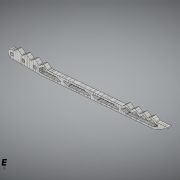
# Autodesk Inventor part: カウンター短
Saved by Autodesk Inventor 2020 (Build 240168000, 168)
## iProperties
Created: 2019-11-14
Part Number: カウンター短
Material: アルミニウム 7075
Document SubType Name: Modeling
Designer: tanjihayato
Density: 2.81 g/cm^3
Appearance: サテン - ブラシ仕上げ 重厚
Mass: 25.3635 g
Surface Area: 57.9543 cm^2
Volume: 9.02615 cm^3
Author: tanjihayato
Autodesk Inventor part; units mm, degrees
ref_plane "YZ Plane" through (0, 0, 0) normal (1, 0, 0) x (0, 1, 0)
ref_plane "XZ Plane" through (0, 0, 0) normal (0, 1, 0) x (-1, 0, 0)
ref_plane "XY Plane" through (0, 0, 0) normal (0, 0, 1) x (1, 0, 0)
sketch "スケッチ1" plane through (0, 0, 0) normal (0, 0, 1) x (1, 0, 0)
  circle A0 centre (0, 0) radius 2
  circle A1 centre (15, 0) radius 2
  arc A2 (0, 5) -> (0, -5) centre (0, 0) ccw
  line L0 (0, 5) -> (35, 5)
  line L1 (23.9629, -5) -> (0, -5)
  line L2 (23.9629, -5) -> (170.722, 7.8398)
  line L3 (170.722, 7.8398) -> (190, 18.5607)
  line L4 (190, 18.5607) -> (35, 5)
  line L5 (170.722, 7.8398) -> (-114.4599, -150.7571)
  dimension "d0" = 4
  dimension "d1" = 4
  dimension "d2" = 15
  dimension "d3" = 3
  dimension "d11" = 175
  dimension "d12" = 9
  dimension "d13" = 175
  dimension "d14" = 35
  constraints: 12 end point, 3 centre point, 2 horizontal, 2 point on circle, 2 tangent, 1 coincident, 1 collinear, 1 horizontal alignment, 1 parallel
  measures "d0" diameter of A0
  measures "d1" diameter of A1
  measures "d2" distance of A1.centre point (0, 0)
  measures "d3" radial gap between concentric circles of A0 A2
  measures "d11" angle of L1 L2
  measures "d12" distance between parallel lines of L2 L4
  measures "d13" horizontal distance of A1.centre L3.end
  measures "d14" distance of L0.start L0.end
extrude "押し出し1" add sketch "スケッチ1" along normal blind 5
sketch "スケッチ2" plane through (0, 0, 5) normal (0, 0, 1) x (1, 0, 0)
  circle A0 centre (15, 0) radius 2 projected
  circle A1 centre (0, 0) radius 2 projected
  arc A2 (0, 5) -> (0, -5) centre (0, 0) ccw projected
  line L0 (0, -5) -> (23.9629, -5) projected
  line L1 (35, 5) -> (0, 5) projected
  arc A3 (0, 5) -> (0, -5) centre (0, 0) ccw projected
  line L2 (-2.9156, 4.0619) -> (3.964, 9)
  line L3 (3.964, 9) -> (9.5368, 5)
  line L4 (9.5368, 5) -> (15.1095, 9)
  line L5 (15.1095, 9) -> (20.6823, 5)
  line L6 (20.6823, 5) -> (26.255, 9)
  line L7 (26.255, 9) -> (31.8278, 5)
  line L8 (-14.2455, 9) -> (62.2851, 9) construction
  line L9 (35, 5) -> (0, 5) projected
  line L10 (23.9629, -5) -> (170.722, 7.8398) projected
  line L11 (170.722, 7.8398) -> (190, 18.5607) projected
  line L12 (190, 18.5607) -> (35, 5) projected
  line L13 (139.8765, 14.1755) -> (145.0794, 18.646)
  line L14 (145.0794, 18.646) -> (150.9795, 15.1469)
  line L15 (150.9795, 15.1469) -> (156.1825, 19.6174)
  line L16 (156.1825, 19.6174) -> (162.0826, 16.1183)
  line L17 (162.0826, 16.1183) -> (167.2855, 20.5888)
  line L18 (167.2855, 20.5888) -> (173.1857, 17.0897)
  line L19 (128.4528, 17.1913) -> (164.3237, 20.3296)
  line L20 (190, 18.5607) -> (35, 5) projected
  dimension "d6" = 144.33
  dimension "d7" = 144.33
  dimension "d15" = 4
  dimension "d16" = 4
  dimension "d17" = 144.33
  dimension "d18" = 144.33
  constraints: 28 end point, 13 point on line, 9 parallel, 1 horizontal, 1 point on circle, 1 tangent
  measures "d6" angle of L8 L3
  measures "d7" angle of L8 L2
  measures "d15" distance between parallel lines of L1 L8
  measures "d16" distance between parallel lines of L19 L12
  measures "d17" angle of L19 L14
  measures "d18" angle of L19 L13
extrude "押し出し2" add sketch "スケッチ2" against normal blind 5 contours A2 L2 L3 L1 | L4 L5 L1 | L6 L7 L1 | L13 L14 L12 | L12 L17 L18 | L15 L16 L12
fillet "フィレット2" radius 0.5 1 edges at (190, 18.5607, 2.5)
sketch "スケッチ3" plane through (0, 0, 5) normal (0, 0, 1) x (1, 0, 0)
  arc A0 (187.9512, 17.4214) -> (187.6646, 18.3564) centre (187.7082, 17.8583) ccw projected
  line L0 (187.6646, 18.3564) -> (173.1857, 17.0897) projected
  line L1 (173.1857, 17.0897) -> (167.2855, 20.5888) projected
  line L2 (167.2855, 20.5888) -> (162.0826, 16.1183) projected
  line L3 (162.0826, 16.1183) -> (156.1825, 19.6174) projected
  line L4 (156.1825, 19.6174) -> (150.9795, 15.1469) projected
  line L5 (150.9795, 15.1469) -> (145.0794, 18.646) projected
  line L6 (145.0794, 18.646) -> (139.8765, 14.1755) projected
  line L7 (139.8765, 14.1755) -> (35, 5) projected
  line L8 (35, 5) -> (31.8278, 5) projected
  line L9 (31.8278, 5) -> (26.255, 9) projected
  line L10 (26.255, 9) -> (20.6823, 5) projected
  line L11 (20.6823, 5) -> (15.1095, 9) projected
  line L12 (15.1095, 9) -> (9.5368, 5) projected
  line L13 (9.5368, 5) -> (3.964, 9) projected
  line L14 (3.964, 9) -> (-2.9156, 4.0619) projected
  arc A1 (-2.9156, 4.0619) -> (0, -5) centre (0, 0) ccw projected
  line L15 (0, -5) -> (23.9629, -5) projected
  line L16 (23.9629, -5) -> (170.722, 7.8398) projected
  line L17 (170.722, 7.8398) -> (187.9512, 17.4214) projected
  circle A2 centre (15, 0) radius 2 projected
  circle A3 centre (0, 0) radius 2 projected
  line L18 (35.1092, 2.5) -> (140.8957, 11.7551)
  line L19 (140.8957, 11.7551) -> (145.3476, 15.5803)
  line L20 (145.3476, 15.5803) -> (151.2478, 12.0813)
  line L21 (151.2478, 12.0813) -> (156.4507, 16.5517)
  line L22 (156.4507, 16.5517) -> (162.3508, 13.0527)
  line L23 (162.3508, 13.0527) -> (167.5537, 17.5231)
  line L24 (167.5537, 17.5231) -> (172.6023, 14.5291)
  line L25 (172.6023, 14.5291) -> (178.5409, 15.0487)
  line L26 (178.5409, 15.0487) -> (169.9729, 10.2838)
  line L27 (169.9729, 10.2838) -> (23.8537, -2.5)
  line L28 (23.8537, -2.5) -> (0, -2.5)
  arc A4 (-1.4578, 2.031) -> (0, -2.5) centre (0, 0) ccw
  line L29 (-1.4578, 2.031) -> (3.964, 5.9227)
  line L30 (3.964, 5.9227) -> (9.5368, 1.9227)
  line L31 (9.5368, 1.9227) -> (15.1095, 5.9227)
  line L32 (15.1095, 5.9227) -> (20.6823, 1.9227)
  line L33 (20.6823, 1.9227) -> (26.255, 5.9227)
  line L34 (26.255, 5.9227) -> (31.0234, 2.5)
  line L35 (31.0234, 2.5) -> (35.1092, 2.5)
  circle A5 centre (15, 0) radius 5.9987
  line L36 (41.5791, 3.0661) -> (52.8759, 0.0391)
  line L37 (58.7012, 0.5488) -> (47.4045, 3.5757)
  line L38 (79.444, 6.3788) -> (90.7407, 3.3518)
  line L39 (96.566, 3.8615) -> (85.2693, 6.8884)
  line L40 (128.6055, 6.6646) -> (117.3088, 9.6915)
  line L41 (134.4308, 7.1742) -> (123.1341, 10.2012)
  point P0 (20.453, -2.5)
  dimension "d20" = 2.5
  dimension "d25" = 2
  dimension "d26" = 2
  dimension "d27" = 2
  dimension "d28" = 11
  dimension "d29" = 11
  dimension "d30" = 20
  constraints: 48 end point, 12 point on line, 5 parallel, 2 point on circle, 1 centre point, 21 other
  measures "d20" distance between parallel lines of L7 L18
  measures "d25" distance between parallel lines of L36 L37
  measures "d26" distance between parallel lines of L38 L39
  measures "d27" distance between parallel lines of L40 L41
  measures "d28" distance between parallel lines of L40 L39
  measures "d29" distance between parallel lines of L37 L38
  measures "d30" angle of L27 L40
extrude "押し出し3" cut sketch "スケッチ3" against normal blind 4 contours A5 L33 L34 L35 L18 L36 L27 L28 | L37 L18 L38 L27 | L39 L18 L40 L27 | L41 L18 L19 L20 L21 L22 L23 L24 L25 L26 L27
fillet "フィレット3" radius 1 25 edges at (20.453, -2.5, 3) (20.6823, 1.9227, 3) (26.255, 5.9227, 3) (31.0234, 2.5, 3) (140.8957, 11.7551, 3) (145.3476, 15.5803, 3) (151.2478, 12.0813, 3) (156.4507, 16.5517, 3) (162.3508, 13.0527, 3) (167.5537, 17.5231, 3) (172.6023, 14.5291, 3) (178.5409, 15.0487, 3) (169.9729, 10.2838, 3) (41.5791, 3.0661, 3) (52.8759, 0.0391, 3) (47.4045, 3.5757, 3) (58.7012, 0.5488, 3) (96.566, 3.8615, 3) (90.7407, 3.3518, 3) (85.2693, 6.8884, 3) (79.444, 6.3788, 3) (117.3088, 9.6915, 3) (128.6055, 6.6646, 3) (123.1341, 10.2012, 3) (134.4308, 7.1742, 3)
sketch "スケッチ4" plane through (0, 0, 5) normal (0, 0, 1) x (1, 0, 0)
  circle A0 centre (0, 0) radius 2 projected
  circle A1 centre (15, 0) radius 2 projected
  arc A2 (187.9512, 17.4214) -> (187.6646, 18.3564) centre (187.7082, 17.8583) ccw projected
  line L0 (187.6646, 18.3564) -> (173.1857, 17.0897) projected
  line L1 (173.1857, 17.0897) -> (167.2855, 20.5888) projected
  line L2 (167.2855, 20.5888) -> (162.0826, 16.1183) projected
  line L3 (162.0826, 16.1183) -> (156.1825, 19.6174) projected
  line L4 (156.1825, 19.6174) -> (150.9795, 15.1469) projected
  line L5 (150.9795, 15.1469) -> (145.0794, 18.646) projected
  line L6 (145.0794, 18.646) -> (139.8765, 14.1755) projected
  line L7 (139.8765, 14.1755) -> (35, 5) projected
  line L8 (35, 5) -> (31.8278, 5) projected
  line L9 (31.8278, 5) -> (26.255, 9) projected
  line L10 (26.255, 9) -> (20.6823, 5) projected
  line L11 (20.6823, 5) -> (15.1095, 9) projected
  line L12 (15.1095, 9) -> (9.5368, 5) projected
  line L13 (9.5368, 5) -> (3.964, 9) projected
  line L14 (3.964, 9) -> (-2.9156, 4.0619) projected
  arc A3 (-2.9156, 4.0619) -> (0, -5) centre (0, 0) ccw projected
  line L15 (0, -5) -> (23.9629, -5) projected
  line L16 (23.9629, -5) -> (170.722, 7.8398) projected
  line L17 (170.722, 7.8398) -> (187.9512, 17.4214) projected
  arc A4 (172.3256, 14.6932) -> (172.9228, 14.5571) centre (172.8357, 15.5533) ccw projected
  line L18 (172.9228, 14.5571) -> (173.8702, 14.64) projected
  arc A5 (174.4433, 12.7699) -> (173.8702, 14.64) centre (173.9573, 13.6438) ccw projected
  line L19 (174.4433, 12.7699) -> (170.1593, 10.3874) projected
  arc A6 (169.7605, 10.2652) -> (170.1593, 10.3874) centre (169.6733, 11.2614) ccw projected
  line L20 (169.7605, 10.2652) -> (134.6065, 7.1896) projected
  arc A7 (134.2605, 7.2199) -> (134.6065, 7.1896) centre (134.5193, 8.1858) ccw projected
  line L21 (134.2605, 7.2199) -> (128.6122, 8.7334) projected
  arc A8 (128.7838, 10.6955) -> (128.6122, 8.7334) centre (128.871, 9.6993) ccw projected
  line L22 (128.7838, 10.6955) -> (140.5751, 11.7271) projected
  arc A9 (140.5751, 11.7271) -> (141.1397, 11.9648) centre (140.488, 12.7233) ccw projected
  line L23 (141.1397, 11.9648) -> (144.8032, 15.1126) projected
  arc A10 (145.965, 15.2142) -> (144.8032, 15.1126) centre (145.4549, 14.3541) ccw projected
  line L24 (145.965, 15.2142) -> (150.6304, 12.4474) projected
  arc A11 (150.6304, 12.4474) -> (151.7922, 12.549) centre (151.1405, 13.3075) ccw projected
  line L25 (151.7922, 12.549) -> (155.9063, 16.084) projected
  arc A12 (157.068, 16.1856) -> (155.9063, 16.084) centre (156.558, 15.3255) ccw projected
  line L26 (157.068, 16.1856) -> (161.7335, 13.4188) projected
  arc A13 (161.7335, 13.4188) -> (162.8952, 13.5204) centre (162.2435, 14.2789) ccw projected
  line L27 (162.8952, 13.5204) -> (167.0093, 17.0554) projected
  arc A14 (168.1711, 17.157) -> (167.0093, 17.0554) centre (167.661, 16.2969) ccw projected
  line L28 (168.1711, 17.157) -> (172.3256, 14.6932) projected
  line L29 (79.6143, 6.3332) -> (85.2626, 4.8197) projected
  arc A15 (85.091, 2.8576) -> (85.2626, 4.8197) centre (85.0038, 3.8538) ccw projected
  line L30 (85.091, 2.8576) -> (58.8769, 0.5641) projected
  arc A16 (58.5309, 0.5944) -> (58.8769, 0.5641) centre (58.7897, 1.5603) ccw projected
  line L31 (58.5309, 0.5944) -> (52.8825, 2.1079) projected
  arc A17 (53.0542, 4.07) -> (52.8825, 2.1079) centre (53.1414, 3.0738) ccw projected
  line L32 (53.0542, 4.07) -> (79.2683, 6.3634) projected
  arc A18 (79.6143, 6.3332) -> (79.2683, 6.3634) centre (79.3555, 5.3672) ccw projected
  arc A19 (30.762, 2.6876) -> (31.3451, 2.5) centre (31.3451, 3.5) ccw projected
  line L33 (31.3451, 2.5) -> (35.1092, 2.5) projected
  line L34 (35.1092, 2.5) -> (41.4035, 3.0507) projected
  arc A20 (41.7495, 3.0204) -> (41.4035, 3.0507) centre (41.4906, 2.0545) ccw projected
  line L35 (41.7495, 3.0204) -> (47.3978, 1.5069) projected
  arc A21 (47.2262, -0.4552) -> (47.3978, 1.5069) centre (47.139, 0.541) ccw projected
  line L36 (47.2262, -0.4552) -> (23.8537, -2.5) projected
  line L37 (23.8537, -2.5) -> (21.8361, -2.5) projected
  arc A22 (20.8593, -1.2857) -> (21.8361, -2.5) centre (21.8361, -1.5) ccw projected
  arc A23 (20.8593, -1.2857) -> (20.8561, 1.3004) centre (15, 0) ccw projected
  arc A24 (21.2492, 2.3296) -> (20.8561, 1.3004) centre (21.8323, 1.5172) ccw projected
  line L38 (21.2492, 2.3296) -> (25.6719, 5.5041) projected
  arc A25 (26.8381, 5.5041) -> (25.6719, 5.5041) centre (26.255, 4.6917) ccw projected
  line L39 (26.8381, 5.5041) -> (30.762, 2.6876) projected
  line L40 (122.9558, 6.1703) -> (96.7417, 3.8769) projected
  arc A26 (96.3957, 3.9071) -> (96.7417, 3.8769) centre (96.6545, 4.8731) ccw projected
  line L41 (96.3957, 3.9071) -> (90.7474, 5.4206) projected
  arc A27 (90.919, 7.3827) -> (90.7474, 5.4206) centre (91.0062, 6.3865) ccw projected
  line L42 (90.919, 7.3827) -> (117.1331, 9.6762) projected
  arc A28 (117.4791, 9.6459) -> (117.1331, 9.6762) centre (117.2203, 8.68) ccw projected
  line L43 (117.4791, 9.6459) -> (123.1275, 8.1324) projected
  arc A29 (122.9558, 6.1703) -> (123.1275, 8.1324) centre (122.8686, 7.1665) ccw projected
  line L44 (0, -5) -> (-15, -5)
  circle A30 centre (-15, 0) radius 2
  circle A31 centre (-15, 0) radius 5
  line L45 (-1.6087, 5) -> (-7.1814, 9)
  line L46 (-7.1814, 9) -> (-12.7542, 5)
  line L47 (9.5368, 5) -> (3.964, 9) projected
  line L48 (-12.7542, 5) -> (-15, 5)
  line L49 (3.964, 9) -> (-17.5463, 9) construction
  dimension "d31" = 4
  dimension "d32" = 3
  dimension "d33" = 15
  constraints: 10 end point, 3 horizontal, 3 point on line, 2 centre point, 2 parallel, 2 point on circle, 2 tangent
  measures "d31" diameter of A30
  measures "d32" radial gap between concentric circles of A30 A31
  measures "d33" distance of A30.centre point (0, 0)
extrude "押し出し4" add sketch "スケッチ4" against normal blind 5 contours L44 A31 L48 L46 L45 L14 A3 | A31
sketch "スケッチ5" plane through (0, 0, 5) normal (0, 0, 1) x (1, 0, 0)
  circle A0 centre (-15, 0) radius 2 projected
  circle A1 centre (0, 0) radius 2 projected
  circle A2 centre (15, 0) radius 2 projected
  arc A3 (187.9512, 17.4214) -> (187.6646, 18.3564) centre (187.7082, 17.8583) ccw projected
  line L0 (187.6646, 18.3564) -> (173.1857, 17.0897) projected
  line L1 (173.1857, 17.0897) -> (167.2855, 20.5888) projected
  line L2 (167.2855, 20.5888) -> (162.0826, 16.1183) projected
  line L3 (162.0826, 16.1183) -> (156.1825, 19.6174) projected
  line L4 (156.1825, 19.6174) -> (150.9795, 15.1469) projected
  line L5 (150.9795, 15.1469) -> (145.0794, 18.646) projected
  line L6 (145.0794, 18.646) -> (139.8765, 14.1755) projected
  line L7 (139.8765, 14.1755) -> (35, 5) projected
  line L8 (35, 5) -> (31.8278, 5) projected
  line L9 (31.8278, 5) -> (26.255, 9) projected
  line L10 (26.255, 9) -> (20.6823, 5) projected
  line L11 (20.6823, 5) -> (15.1095, 9) projected
  line L12 (15.1095, 9) -> (9.5368, 5) projected
  line L13 (9.5368, 5) -> (3.964, 9) projected
  line L14 (3.964, 9) -> (-1.6087, 5) projected
  line L15 (-1.6087, 5) -> (-7.1814, 9) projected
  line L16 (-7.1814, 9) -> (-12.7542, 5) projected
  line L17 (-12.7542, 5) -> (-15, 5) projected
  arc A4 (-15, 5) -> (-15, -5) centre (-15, 0) ccw projected
  line L18 (-15, -5) -> (23.9629, -5) projected
  line L19 (23.9629, -5) -> (170.722, 7.8398) projected
  line L20 (170.722, 7.8398) -> (187.9512, 17.4214) projected
  arc A5 (172.3256, 14.6932) -> (172.9228, 14.5571) centre (172.8357, 15.5533) ccw projected
  line L21 (172.9228, 14.5571) -> (173.8702, 14.64) projected
  arc A6 (174.4433, 12.7699) -> (173.8702, 14.64) centre (173.9573, 13.6438) ccw projected
  line L22 (174.4433, 12.7699) -> (170.1593, 10.3874) projected
  arc A7 (169.7605, 10.2652) -> (170.1593, 10.3874) centre (169.6733, 11.2614) ccw projected
  line L23 (169.7605, 10.2652) -> (134.6065, 7.1896) projected
  arc A8 (134.2605, 7.2199) -> (134.6065, 7.1896) centre (134.5193, 8.1858) ccw projected
  line L24 (134.2605, 7.2199) -> (128.6122, 8.7334) projected
  arc A9 (128.7838, 10.6955) -> (128.6122, 8.7334) centre (128.871, 9.6993) ccw projected
  line L25 (128.7838, 10.6955) -> (140.5751, 11.7271) projected
  arc A10 (140.5751, 11.7271) -> (141.1397, 11.9648) centre (140.488, 12.7233) ccw projected
  line L26 (141.1397, 11.9648) -> (144.8032, 15.1126) projected
  arc A11 (145.965, 15.2142) -> (144.8032, 15.1126) centre (145.4549, 14.3541) ccw projected
  line L27 (145.965, 15.2142) -> (150.6304, 12.4474) projected
  arc A12 (150.6304, 12.4474) -> (151.7922, 12.549) centre (151.1405, 13.3075) ccw projected
  line L28 (151.7922, 12.549) -> (155.9063, 16.084) projected
  arc A13 (157.068, 16.1856) -> (155.9063, 16.084) centre (156.558, 15.3255) ccw projected
  line L29 (157.068, 16.1856) -> (161.7335, 13.4188) projected
  arc A14 (161.7335, 13.4188) -> (162.8952, 13.5204) centre (162.2435, 14.2789) ccw projected
  line L30 (162.8952, 13.5204) -> (167.0093, 17.0554) projected
  arc A15 (168.1711, 17.157) -> (167.0093, 17.0554) centre (167.661, 16.2969) ccw projected
  line L31 (168.1711, 17.157) -> (172.3256, 14.6932) projected
  line L32 (79.6143, 6.3332) -> (85.2626, 4.8197) projected
  arc A16 (85.091, 2.8576) -> (85.2626, 4.8197) centre (85.0038, 3.8538) ccw projected
  line L33 (85.091, 2.8576) -> (58.8769, 0.5641) projected
  arc A17 (58.5309, 0.5944) -> (58.8769, 0.5641) centre (58.7897, 1.5603) ccw projected
  line L34 (58.5309, 0.5944) -> (52.8825, 2.1079) projected
  arc A18 (53.0542, 4.07) -> (52.8825, 2.1079) centre (53.1414, 3.0738) ccw projected
  line L35 (53.0542, 4.07) -> (79.2683, 6.3634) projected
  arc A19 (79.6143, 6.3332) -> (79.2683, 6.3634) centre (79.3555, 5.3672) ccw projected
  arc A20 (30.762, 2.6876) -> (31.3451, 2.5) centre (31.3451, 3.5) ccw projected
  line L36 (31.3451, 2.5) -> (35.1092, 2.5) projected
  line L37 (35.1092, 2.5) -> (41.4035, 3.0507) projected
  arc A21 (41.7495, 3.0204) -> (41.4035, 3.0507) centre (41.4906, 2.0545) ccw projected
  line L38 (41.7495, 3.0204) -> (47.3978, 1.5069) projected
  arc A22 (47.2262, -0.4552) -> (47.3978, 1.5069) centre (47.139, 0.541) ccw projected
  line L39 (47.2262, -0.4552) -> (23.8537, -2.5) projected
  line L40 (23.8537, -2.5) -> (21.8361, -2.5) projected
  arc A23 (20.8593, -1.2857) -> (21.8361, -2.5) centre (21.8361, -1.5) ccw projected
  arc A24 (20.8593, -1.2857) -> (20.8561, 1.3004) centre (15, 0) ccw projected
  arc A25 (21.2492, 2.3296) -> (20.8561, 1.3004) centre (21.8323, 1.5172) ccw projected
  line L41 (21.2492, 2.3296) -> (25.6719, 5.5041) projected
  arc A26 (26.8381, 5.5041) -> (25.6719, 5.5041) centre (26.255, 4.6917) ccw projected
  line L42 (26.8381, 5.5041) -> (30.762, 2.6876) projected
  line L43 (122.9558, 6.1703) -> (96.7417, 3.8769) projected
  arc A27 (96.3957, 3.9071) -> (96.7417, 3.8769) centre (96.6545, 4.8731) ccw projected
  line L44 (96.3957, 3.9071) -> (90.7474, 5.4206) projected
  arc A28 (90.919, 7.3827) -> (90.7474, 5.4206) centre (91.0062, 6.3865) ccw projected
  line L45 (90.919, 7.3827) -> (117.1331, 9.6762) projected
  arc A29 (117.4791, 9.6459) -> (117.1331, 9.6762) centre (117.2203, 8.68) ccw projected
  line L46 (117.4791, 9.6459) -> (123.1275, 8.1324) projected
  arc A30 (122.9558, 6.1703) -> (123.1275, 8.1324) centre (122.8686, 7.1665) ccw projected
  line L47 (139.8765, 14.1755) -> (133.9763, 17.6746)
  line L48 (133.9763, 17.6746) -> (128.7734, 13.2041)
  line L49 (145.0794, 18.646) -> (120.5189, 16.4972)
  line L50 (150.9795, 15.1469) -> (145.0794, 18.646) projected
  line L51 (128.7838, 10.6955) -> (140.5751, 11.7271) projected
  line L52 (140.1447, 11.1099) -> (134.2445, 14.609)
  line L53 (134.2445, 14.609) -> (129.3917, 10.4393)
  line L54 (141.1397, 11.9648) -> (140.1447, 11.1099)
  point P0 (139.2931, 11.6149)
  point P1 (133.0444, 13.5778)
  point P2 (135.6055, 13.8018)
  point P3 (129.7926, 10.7837)
  dimension "d36" = 2.5
  dimension "d37" = 2.5
  constraints: 12 end point, 4 parallel, 3 point on line, 1 collinear
  measures "d36" distance between parallel lines of L52 L47
  measures "d37" distance between parallel lines of L48 L53
extrude "押し出し5" add sketch "スケッチ5" against normal blind 5 contours L7 L52 L53 L48 L47 | L7 L53 L52 | L25 A10 L54 L52
extrude "押し出し6" cut sketch "スケッチ5" against normal blind 4 contours L52 L25 L53 L7 | L7 L53 L52
fillet "フィレット4" radius 1 3 edges at (140.1447, 11.1099, 3) (134.2445, 14.609, 3) (129.7926, 10.7837, 3)
equation "\"d7\" = d6"
equation "\"d17\" = d6"
equation "\"d18\" = d17"
